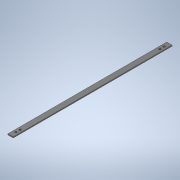
# Autodesk Inventor part: listwa_weglowa
Saved by Autodesk Inventor 2021 (Build 250183000, 183)
## iProperties
Created: 2021-05-05
Part Number: listwa_weglowa
Material: Ogólny
Document SubType Name: Modeling
Designer: kriso
Density: 1 g/cm^3
Appearance: Odlew czarny
Author: kriso
Autodesk Inventor part; units mm, degrees
ref_plane "YZ Plane" through (0, 0, 0) normal (1, 0, 0) x (0, 1, 0)
ref_plane "XZ Plane" through (0, 0, 0) normal (0, 1, 0) x (-1, 0, 0)
ref_plane "XY Plane" through (0, 0, 0) normal (0, 0, 1) x (1, 0, 0)
sketch "Szkic1" plane through (0, 0, 0) normal (0, 1, 0) x (-1, 0, 0)
  line L0 (-2.5, 75) -> (2.5, 75)
  line L1 (2.5, 75) -> (2.5, -75)
  line L2 (2.5, -75) -> (-2.5, -75)
  line L3 (-2.5, -75) -> (-2.5, 75)
  line L4 (-2.5, 75) -> (2.5, -75) construction
  line L5 (2.5, 75) -> (-2.5, -75) construction
  line L6 (0, 75) -> (0, 70) construction
  circle A0 centre (0, 70) radius 1
  line L7 (0, 70) -> (0, 66) construction
  circle A1 centre (0, 66) radius 1
  line L8 (0, -75) -> (0, -70) construction
  circle A2 centre (0, -70) radius 1
  line L9 (0, -70) -> (0, -66) construction
  circle A3 centre (0, -66) radius 1
  point P0 (0, 0)
  dimension "d0" = 5
  dimension "d1" = 150
  dimension "d2" = 5
  dimension "d3" = 2
  dimension "d4" = 4
  dimension "d5" = 2
  dimension "d6" = 5
  dimension "d7" = 2
  dimension "d8" = 4
  dimension "d9" = 2
  constraints: 20 end point, 4 centre point, 4 coincident, 4 midpoint, 4 vertical, 2 parallel, 1 horizontal, 1 perpendicular
  measures "d0" distance of L1.end L2.end
  measures "d1" distance of L0.end L1.end
  measures "d2" distance of L6.start L6.end
  measures "d3" diameter of A0
  measures "d4" distance of L7.start L7.end
  measures "d5" diameter of A1
  measures "d6" distance of L8.start L8.end
  measures "d7" diameter of A2
  measures "d8" distance of L9.start L9.end
  measures "d9" diameter of A3
extrude "Wyciągnięcie proste1" add sketch "Szkic1" along normal blind 1
